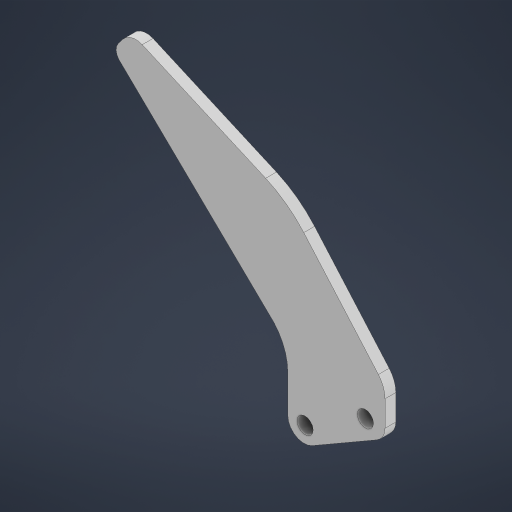
# Autodesk Inventor part: Claw Tip
Saved by Autodesk Inventor 2023 (Build 270158000, 158)
## iProperties
Created: 2023-04-12
Part Number: Claw Tip
Material: Generic
Document SubType Name: Modeling
Designer: vatdu
Density: 1 g/cm^3
Appearance: Default
Author: vatdu
Autodesk Inventor part; units mm, degrees
ref_plane "YZ Plane" through (0, 0, 0) normal (1, 0, 0) x (0, 1, 0)
ref_plane "XZ Plane" through (0, 0, 0) normal (0, 1, 0) x (-1, 0, 0)
ref_plane "XY Plane" through (0, 0, 0) normal (0, 0, 1) x (1, 0, 0)
sketch "Sketch1" plane through (0, 0, 0) normal (0, 0, 1) x (1, 0, 0)
  line L0 (0, 0) -> (18, 0)
  line L1 (18, 0) -> (18, 30)
  line L2 (18, 30) -> (0, 30)
  line L3 (0, 30) -> (0, 0)
  line L4 (0, 0) -> (18, 10.3923)
  line L5 (0, 0) -> (20.7846, 0) construction
  dimension "d0" = 18
  dimension "d1" = 30
  dimension "d2" = 30
  constraints: 12 end point, 2 horizontal, 2 parallel, 1 equal length, 1 perpendicular, 1 point on line
  measures "d0" distance of L2.end L1.end
  measures "d1" distance of L1.end L0.end
  measures "d2" angle of L5 L4
extrude "Extrusion1" add sketch "Sketch1" along normal blind 2 contours L3 L2 L1 L4
fillet "Fillet1" radius 3 2 edges at (0, 0, 1) (18, 10.3923, 1)
sketch "Sketch2" plane through (0, 0, 2) normal (0, 0, 1) x (1, 0, 0)
  arc A0 (0, 5.1962) -> (4.5, 2.5981) centre (3, 5.1962) ccw projected
  arc A1 (16.5, 9.5263) -> (18, 12.1244) centre (15, 12.1244) ccw projected
  line L0 (4.5, 2.5981) -> (16.5, 9.5263) projected
  line L1 (10.5, 6.0622) -> (8.7793, 8.5196)
  line L2 (10.5, 6.0622) -> (13.5, 6.0622) construction
  line L3 (8.7793, 8.5196) -> (3.1932, 5.1962)
  line L4 (3.1932, 5.1962) -> (14.3654, 11.8431)
  circle A2 centre (3.1932, 5.1962) radius 1.5
  circle A3 centre (14.3654, 11.8431) radius 1.5
  point P0 (0, 0)
  dimension "d8" = 3
  dimension "d9" = 125
  dimension "d10" = 6.5
  dimension "d11" = 13
  dimension "d12" = 3
  dimension "d13" = 3
  constraints: 8 end point, 2 centre point, 2 coincident, 1 equal length, 1 horizontal, 1 midpoint, 1 point on line
  measures "d8" distance of L1.start L1.end
  measures "d9" angle of L2 L1
  measures "d10" distance of L1.end L3.end
  measures "d11" distance of L3.end L4.end
  measures "d12" diameter of A2
  measures "d13" diameter of A3
extrude "Extrusion2" cut sketch "Sketch2" against normal blind 2
sketch "Sketch3" plane through (0, 0, 2) normal (0, 0, 1) x (1, 0, 0)
  line L0 (18, 12.1244) -> (18, 30) projected
  line L1 (18, 30) -> (4.0584, 13.3851)
  line L2 (18, 30) -> (39.6893, 30) construction
  line L3 (4.0584, 13.3851) -> (-34.2438, 45.5244)
  line L4 (-34.2438, 45.5244) -> (-20.9174, 62.6556)
  line L5 (-20.9174, 62.6556) -> (18, 30)
  point P0 (0, 0)
  dimension "d16" = 130
  dimension "d17" = 50
  dimension "d18" = 90
  constraints: 10 end point, 1 equal length, 1 horizontal, 1 parallel, 1 perpendicular
  measures "d16" angle of L1 L2
  measures "d17" distance of L1.end L3.end
  measures "d18" angle of L1 L3
extrude "Extrusion3" cut sketch "Sketch3" against normal blind 2
extrude "Extrusion4" add sketch "Sketch3" against normal blind 2
fillet "Fillet2" radius 10 2 edges at (18, 30, 1) (0, 16.7905, 1)
chamfer "Chamfer1" distance 5 distance2 40 1 edges at (-20.9174, 62.6556, 1) measured on face at (-25.3595, 56.9452, 1.3333)
fillet "Fillet3" radius 20 1 edges at (9.7244, 36.9441, 1)
sketch "Sketch4" plane through (0, 0, 2) normal (0, 0, 1) x (1, 0, 0)
  line L0 (-23.9874, 58.7091) -> (8.6742, 37.6221) projected
  line L1 (-7.6566, 48.1656) -> (18, 18.7306)
  line L2 (18, 12.1244) -> (18, 25.3369) projected
  line L3 (-7.6566, 48.1656) -> (3.9893, 54.5621)
  line L4 (3.9893, 54.5621) -> (27.8287, 24.1291)
  line L5 (27.8287, 24.1291) -> (18, 18.7306)
  point P0 (0, 0)
  constraints: 8 end point, 3 midpoint, 1 parallel
extrude "Extrusion5" cut sketch "Sketch4" against normal blind 2
fillet "Fillet4" radius 5 1 edges at (18, 18.7306, 1)
sketch "Sketch5" plane through (0, 0, 2) normal (0, 0, 1) x (1, 0, 0)
  line L0 (16.7692, 20.1427) -> (-7.6566, 48.1656) projected
  line L1 (0, 39.3814) -> (-29.1156, 52.1168)
  line L2 (-34.2438, 45.5244) -> (-23.9874, 58.7091) projected
  line L3 (-29.1156, 52.1168) -> (-28.0652, 63.5725)
  line L4 (-28.0652, 63.5725) -> (-0.6496, 57.8446)
  line L5 (-0.6496, 57.8446) -> (0, 39.3814)
  point P0 (0, 0)
  constraints: 8 end point, 1 midpoint, 1 point on line
extrude "Extrusion6" cut sketch "Sketch5" against normal blind 2
fillet "Fillet5" radius 20 1 edges at (0, 39.3814, 1)
fillet "Fillet6" radius 3 1 edges at (-29.1156, 52.1168, 1)
chamfer "Chamfer2" distance 20 distance2 3 1 edges at (-34.2438, 45.5244, 1) measured on face at (-24.0199, 36.9456, 1.3333)
fillet "Fillet7" radius 2 1 edges at (-32.4018, 47.8923, 1)
sketch "Sketch6" plane through (0, 0, 2) normal (0, 0, 1) x (1, 0, 0)
  line L0 (-31.3011, 46.6491) -> (-18.9229, 32.6687) projected
  arc A0 (0, 12.1274) -> (-3.5721, 19.7878) centre (-10, 12.1274) ccw projected
  line L1 (-31.3011, 46.6491) -> (-3.5721, 19.7878)
  line L2 (-3.5721, 19.7878) -> (-20.8807, 12.1274)
  arc A1 (-31.3823, 49.203) -> (-31.3011, 46.6491) centre (-29.8037, 47.9749) ccw projected
  line L3 (-20.8807, 12.1274) -> (-31.3011, 46.6491)
  point P0 (0, 0)
  constraints: 6 end point
extrude "Extrusion7" cut sketch "Sketch6" against normal blind 10
body "Solid1"
